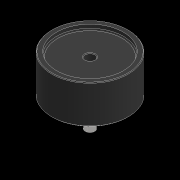
# Autodesk Inventor part: MockupWheel
Saved by Autodesk Inventor 2021 (Build 250183000, 183)
## iProperties
Created: 2021-01-23
Part Number: MockupWheel
Material: Rubber, Silicone
Document SubType Name: Modeling
Designer: Esketitttttt
Density: 1.25 g/cm^3
Appearance: Rubber - Black
Mass: 4054.17 g
Surface Area: 1368.11 cm^2
Volume: 3243.33 cm^3
Author: Esketitttttt
Autodesk Inventor part; units mm, degrees
ref_plane "YZ Plane" through (0, 0, 0) normal (1, 0, 0) x (0, 1, 0)
ref_plane "XZ Plane" through (0, 0, 0) normal (0, 1, 0) x (-1, 0, 0)
ref_plane "XY Plane" through (0, 0, 0) normal (0, 0, 1) x (1, 0, 0)
sketch "Sketch1" plane through (0, 0, 0) normal (0, 1, 0) x (-1, 0, 0)
  circle A0 centre (0, 0) radius 101.6
  circle A1 centre (0, 0) radius 12.7
  dimension "d0" = 203.2
  dimension "d1" = 25.4
  constraints: 2 centre point, 2 coincident
  measures "d0" diameter of A0
  measures "d1" diameter of A1
extrude "Extrusion1" add sketch "Sketch1" along normal blind 101.6
sketch "Sketch2" plane through (0, 0, 0) normal (0, -1, 0) x (1, 0, 0)
  circle A0 centre (0, 0) radius 101.6 projected
  circle A1 centre (0, 0) radius 12.7 projected
extrude "Extrusion2" add sketch "Sketch2" along normal blind 76.2 and the other way blind 50.8 contours A1
sketch "Sketch3" plane through (0, 101.6, 0) normal (0, 1, 0) x (1, 0, 0)
  circle A0 centre (0, 0) radius 101.6 projected
  circle A1 centre (0, 0) radius 12.7 projected
  circle A2 centre (0, 0) radius 88.9
  dimension "d8" = 12.7
  constraints: 1 centre point
  measures "d8" radial gap between concentric circles of A0 A2
extrude "Extrusion3" cut sketch "Sketch3" against normal blind 12.7 contours A2
fillet "Fillet1" radius 3.175 1 edges at (-88.9, 88.9, 0)
fillet "Fillet2" radius 1.5875 3 edges at (101.6, 101.6, 0) (101.6, 0, 0) (12.7, 88.9, 0)
body "Solid1"
